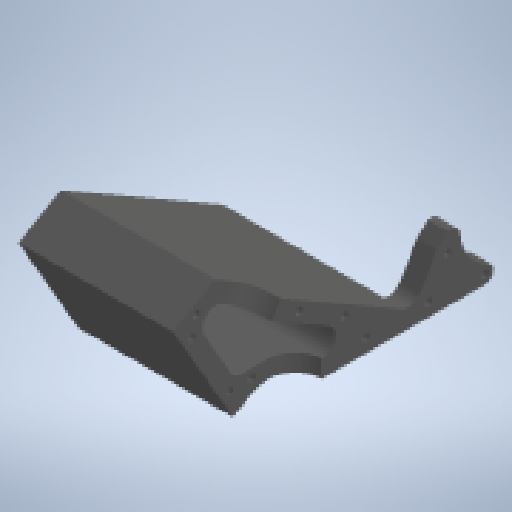
# Autodesk Inventor part: leg_upper_middle_left
Saved by Autodesk Inventor 2024.1 (Build 281209000, 209)
## iProperties
Created: 2024-10-11
Part Number: leg_upper_middle_left
Material: 一般
Document SubType Name: Modeling
Designer: hibik
Density: 1 g/cm^3
Appearance: 既定
Author: hibik
Autodesk Inventor part; units mm, degrees
ref_plane "YZ Plane" through (0, 0, 0) normal (1, 0, 0) x (0, 1, 0)
ref_plane "XZ Plane" through (0, 0, 0) normal (0, 1, 0) x (-1, 0, 0)
ref_plane "XY Plane" through (0, 0, 0) normal (0, 0, 1) x (1, 0, 0)
sketch "スケッチ1" plane through (0, 0, 0) normal (1, 0, 0) x (0, 1, 0)
  line L0 (27, 0) -> (0, 0)
  line L1 (0, 0) -> (0, -65.8723)
  line L2 (0, -65.8723) -> (27, -65.8723)
  line L3 (27, -65.8723) -> (27, -2.1436)
  line L4 (25.9282, 1.8564) -> (7.2963, 34.1277)
  line L5 (7.2963, 34.1277) -> (-16.0863, 20.6277)
  line L6 (-16.0863, 20.6277) -> (0, -7.2346)
  line L7 (0, 19.7654) -> (-4.395, 27.3777)
  circle A0 centre (0, 19.7654) radius 4.25
  circle A1 centre (13.5, -57.0823) radius 4.25
  line L8 (13.5, -65.8723) -> (13.5, -57.0823)
  circle A2 centre (0, 19.7654) radius 13.5
  circle A3 centre (13.5, -57.0823) radius 13.5
  circle A4 centre (0, 19.7654) radius 6
  circle A5 centre (13.5, -57.0823) radius 6
  circle A6 centre (-3, 24.9615) radius 1
  circle A7 centre (-5.7956, 21.3183) radius 1
  circle A8 centre (-5.1962, 16.7654) radius 1
  circle A9 centre (-1.5529, 13.9698) radius 1
  circle A10 centre (3, 14.5692) radius 1
  circle A11 centre (5.7956, 18.2125) radius 1
  circle A12 centre (13.5, -63.0823) radius 1
  circle A13 centre (17.7426, -61.3249) radius 1
  circle A14 centre (19.5, -57.0823) radius 1
  circle A15 centre (17.7426, -52.8396) radius 1
  circle A16 centre (13.5, -51.0823) radius 1
  circle A17 centre (9.2574, -52.8396) radius 1
  circle A18 centre (7.5, -57.0823) radius 1
  circle A19 centre (9.2574, -61.3249) radius 1
  circle A20 centre (5.1962, 22.7654) radius 1
  circle A21 centre (1.5529, 25.5609) radius 1
  line L9 (13.5, -57.0823) -> (50.1936, 6.4729)
  line L10 (13.5, -57.0823) -> (5.7058, -52.5823)
  line L11 (12.2058, -41.3239) -> (-0.7942, -63.8406)
  line L12 (12.2058, -41.3239) -> (3.1125, -36.0739)
  line L13 (3.1125, -36.0739) -> (27, 5.3004)
  line L14 (19.9413, 12.226) -> (-3.4413, -1.274)
  line L15 (3.1125, -36.0739) -> (0, -36.0739)
  arc A22 (27, -2.1436) -> (25.9282, 1.8564) centre (19, -2.1436) ccw
  point P0 (-14.7211, 28.9596)
  point P1 (-3.0298, -41.1381)
  point P2 (23.9702, -41.1381)
  point P3 (8.6616, 42.4596)
  point P4 (25.4699, 2.6502)
  point P5 (0, -57.0823)
  point P6 (10.7369, -43.8681)
  dimension "d11" = 12
  dimension "d12" = 12
  dimension "d4" = 27
  dimension "d5" = 150
  dimension "d6" = 27
  dimension "d7" = 8.79
  dimension "d8" = 100
  dimension "d9" = 8.79
  dimension "d10" = 8.5
  dimension "d13" = 2
  dimension "d14" = 360
  dimension "d15" = 2
  dimension "d16" = 360
  dimension "d17" = 39.4073
  dimension "d18" = 9
  dimension "d19" = 13
  dimension "d20" = 30
  dimension "d22" = 19.5
  dimension "d24" = 16.5
  dimension "d28" = 8
  constraints: 32 end point, 21 centre point, 9 perpendicular, 9 point on line, 8 coincident, 4 tangent, 3 midpoint, 2 parallel, 2 point on circle, 2 vertical alignment, 1 equal radius, 1 horizontal, 1 vertical, 40 other
  measures "d4" distance of L1.end L2.end
  measures "d5" angle of L3 L4
  measures "d6" distance between parallel lines of L6 L4
  measures "d7" distance from line of L5 L7.start
  measures "d8" distance from line of L2 L4.end
  measures "d9" distance of L8.start point (13.5, -57.082)
  measures "d10" diameter of A0
  measures "d13" diameter of A6
  measures "d15" diameter of A12
  measures "d17" distance from line of L0.start L5
  measures "d18" distance from line of L10.end L9
  measures "d19" distance from line of L11.start L10
  measures "d20" angle of L3 L9
  measures "d22" distance from line of L13 L8.end
  measures "d24" distance from line of L14 L7.start
  measures "d28" radius of A22
extrude "押し出し1" add sketch "スケッチ1" along normal blind 35 contours L13 L15 L1 L0 | L0 L1 L6 L14 L4 L13
fillet "フィレット1" radius 8 1 edges at (17.5, 0, -7.2346)
sketch "スケッチ2" plane through (35, 0, 0) normal (1, 0, 0) x (0, 0, -1)
  line L0 (21.5464, 11.5) -> (9.5919, 18.4019) projected
  arc A0 (11.0919, 24) -> (9.5919, 18.4019) centre (11.0919, 21) ccw projected
  line L1 (11.0919, 24) -> (27.0312, 24) projected
  arc A1 (29.6293, 19.5) -> (27.0312, 24) centre (27.0312, 21) ccw projected
  line L2 (29.6293, 19.5) -> (25.6444, 12.5981) projected
  arc A2 (21.5464, 11.5) -> (25.6444, 12.5981) centre (23.0464, 14.0981) ccw projected
  line L3 (-15.2943, 14.7058) -> (-13.324, 15.8433) projected
  arc A3 (-9.226, 14.7452) -> (-13.324, 15.8433) centre (-11.824, 13.2452) ccw projected
  line L4 (-9.226, 14.7452) -> (-1.726, 1.7548) projected
  arc A4 (-2.824, -2.3433) -> (-1.726, 1.7548) centre (-4.324, 0.2548) ccw projected
  line L5 (-2.824, -2.3433) -> (-4.7943, -3.4808) projected
  arc A5 (-9.2878, -0.6865) -> (-4.7943, -3.4808) centre (-6.2943, -0.8827) ccw projected
  arc A6 (-9.2878, -0.6865) -> (-15.1212, 9.4171) centre (-19.7654, 0) ccw projected
  arc A7 (-15.2943, 14.7058) -> (-15.1212, 9.4171) centre (-13.7943, 12.1077) ccw projected
  line L6 (45.8573, 3) -> (37.0726, 3) projected
  arc A8 (35.5726, 3.4019) -> (37.0726, 3) centre (37.0726, 6) ccw projected
  line L7 (35.5726, 3.4019) -> (31.9387, 5.5) projected
  arc A9 (30.8406, 9.5981) -> (31.9387, 5.5) centre (33.4387, 8.0981) ccw projected
  line L8 (30.8406, 9.5981) -> (38.2895, 22.5) projected
  arc A10 (40.8876, 24) -> (38.2895, 22.5) centre (40.8876, 21) ccw projected
  line L9 (40.8876, 24) -> (45.8573, 24) projected
  arc A11 (48.3517, 19.3333) -> (45.8573, 24) centre (45.8573, 21) ccw projected
  arc A12 (48.3517, 19.3333) -> (48.3517, 7.6667) centre (57.0823, 13.5) ccw projected
  arc A13 (45.8573, 3) -> (48.3517, 7.6667) centre (45.8573, 6) ccw projected
  line L10 (-1.1502, 19.9851) -> (16.8406, 9.5981) projected
  arc A14 (15.3406, 4) -> (16.8406, 9.5981) centre (15.3406, 7) ccw projected
  line L11 (15.3406, 4) -> (3.3286, 4) projected
  arc A15 (0.7306, 5.5) -> (3.3286, 4) centre (3.3286, 7) ccw projected
  line L12 (0.7306, 5.5) -> (-5.2619, 15.8792) projected
  arc A16 (-4.1638, 19.9772) -> (-5.2619, 15.8792) centre (-2.6638, 17.3792) ccw projected
  line L13 (-4.1638, 19.9772) -> (-4.1502, 19.9851) projected
  arc A17 (-1.1502, 19.9851) -> (-4.1502, 19.9851) centre (-2.6502, 17.387) ccw projected
  arc A18 (57.3667, 17.7405) -> (59.3483, 18.9706) centre (57.5005, 19.736) ccw projected
  line L14 (59.3483, 18.9706) -> (59.8105, 20.0866) projected
  arc A19 (59.8105, 20.0866) -> (55.1911, 27) centre (55.1911, 22) ccw projected
  line L15 (55.1911, 27) -> (2.1436, 27) projected
  arc A20 (2.1436, 27) -> (-1.8564, 25.9282) centre (2.1436, 19) ccw projected
  line L16 (-1.8564, 25.9282) -> (-24.8776, 12.6369) projected
  arc A21 (-24.8776, 12.6369) -> (-25.4214, 4.34) centre (-22.3776, 8.3068) ccw projected
  line L17 (-25.4214, 4.34) -> (-24.4631, 3.6047) projected
  arc A22 (-24.4631, 3.6047) -> (-22.1319, 3.5302) centre (-23.2456, 5.1914) ccw projected
  arc A23 (-17.8914, -3.8146) -> (-22.1319, 3.5302) centre (-19.7654, 0) ccw projected
  arc A24 (-17.8914, -3.8146) -> (-18.9925, -5.8707) centre (-17.0096, -5.6096) ccw projected
  line L18 (-18.9925, -5.8707) -> (-18.8348, -7.0683) projected
  arc A25 (-18.8348, -7.0683) -> (-11.3776, -10.7458) centre (-13.8776, -6.4156) ccw projected
  line L19 (-11.3776, -10.7458) -> (5.3782, -1.0718) projected
  arc A26 (9.3782, 0) -> (5.3782, -1.0718) centre (9.3782, -8) ccw projected
  line L20 (9.3782, 0) -> (55.1911, 0) projected
  arc A27 (55.1911, 0) -> (59.8105, 6.9134) centre (55.1911, 5) ccw projected
  line L21 (59.8105, 6.9134) -> (59.3483, 8.0294) projected
  arc A28 (59.3483, 8.0294) -> (57.3667, 9.2595) centre (57.5005, 7.264) ccw projected
  arc A29 (57.3667, 17.7405) -> (57.3667, 9.2595) centre (57.0823, 13.5) ccw projected
  circle A30 centre (-22.7654, 5.1962) radius 1 projected
  circle A31 centre (-18.2125, 5.7956) radius 1 projected
  circle A32 centre (-14.5692, 3) radius 1 projected
  circle A33 centre (-13.9698, -1.5529) radius 1 projected
  circle A34 centre (-16.7654, -5.1962) radius 1 projected
  circle A35 centre (57.0823, 19.5) radius 1 projected
  circle A36 centre (52.8396, 17.7426) radius 1 projected
  circle A37 centre (51.0823, 13.5) radius 1 projected
  circle A38 centre (52.8396, 9.2574) radius 1 projected
  circle A39 centre (57.0823, 7.5) radius 1 projected
  circle A40 centre (5.5061, 2) radius 1 projected
  circle A41 centre (10.1981, 15.7425) radius 1 projected
  circle A42 centre (25.3406, 3) radius 1 projected
  circle A43 centre (0.5061, 1.8888) radius 1 projected
  circle A44 centre (20.5464, 9.7679) radius 1 projected
  circle A45 centre (-7.9939, 16.6112) radius 1 projected
  circle A46 centre (-6.8958, 20.7093) radius 1 projected
  point P0 (0, 0)
extrude "押し出し2" cut sketch "スケッチ2" against normal through all contours L10 A14 L11 A15 L12 A16 L13 A17
sketch "スケッチ3" plane through (0, 0, 0) normal (-1, 0, 0) x (0, 0, 1)
  arc A0 (-3.3286, 4) -> (-0.7306, 5.5) centre (-3.3286, 7) ccw projected
  line L0 (-3.3286, 4) -> (-15.3406, 4) projected
  arc A1 (-16.8406, 9.5981) -> (-15.3406, 4) centre (-15.3406, 7) ccw projected
  line L1 (-16.8406, 9.5981) -> (1.1502, 19.9851) projected
  arc A2 (4.1502, 19.9851) -> (1.1502, 19.9851) centre (2.6502, 17.387) ccw projected
  line L2 (4.1502, 19.9851) -> (4.1638, 19.9772) projected
  arc A3 (5.2619, 15.8792) -> (4.1638, 19.9772) centre (2.6638, 17.3792) ccw projected
  line L3 (5.2619, 15.8792) -> (-0.7306, 5.5) projected
  line L4 (-36.0739, 3.1125) -> (2.6502, 25.4699) projected
  line L5 (-36.0739, 0) -> (-36.0739, 3.1125) projected
  line L6 (-9.3782, 0) -> (-36.0739, 0) projected
  arc A4 (-5.3782, -1.0718) -> (-9.3782, 0) centre (-9.3782, -8) ccw projected
  line L7 (-1.274, -3.4413) -> (-5.3782, -1.0718) projected
  line L8 (12.226, 19.9413) -> (-1.274, -3.4413) projected
  line L9 (2.6502, 25.4699) -> (12.226, 19.9413) projected
  line L10 (1.1502, 19.9851) -> (-0.8498, 23.4492)
  line L11 (-6.0459, 20.4492) -> (-4.0459, 16.9851)
  line L12 (-15.3346, 4) -> (-15.3346, 0)
  line L13 (-3.3286, 4) -> (-15.3406, 4) projected
  line L14 (-9.3782, 0) -> (-9.3782, 4)
  point P0 (0, 0)
  point P1 (-9.3346, 4)
  dimension "d33" = 6
  dimension "d34" = 6
  constraints: 8 end point, 6 point on line, 4 perpendicular, 1 midpoint
  measures "d33" distance between parallel lines of L10 L11
  measures "d34" distance from line of point (-9.335, 4) L12
extrude "押し出し3" add sketch "スケッチ3" along normal blind 6 contours L12 L6 L5 L4 L11 L1 A1 L0
fillet "フィレット2" radius 6 2 edges at (0, 18.7171, -5.0459) (0, 2, -15.3346)
sketch "スケッチ4" plane through (-6, 0, 0) normal (-1, 0, 0) x (0, 0, 1)
  arc A0 (-39.4731, 0) -> (-36.875, 4.5) centre (-39.4731, 3) ccw projected
  line L0 (-39.4731, 0) -> (-55.1911, 0) projected
  arc A1 (-59.8105, 6.9134) -> (-55.1911, 0) centre (-55.1911, 5) ccw projected
  line L1 (-59.8105, 6.9134) -> (-59.3483, 8.0294) projected
  arc A2 (-57.3667, 9.2595) -> (-59.3483, 8.0294) centre (-57.5005, 7.264) ccw projected
  arc A3 (-57.3667, 9.2595) -> (-57.3667, 17.7405) centre (-57.0823, 13.5) ccw projected
  arc A4 (-59.3483, 18.9706) -> (-57.3667, 17.7405) centre (-57.5005, 19.736) ccw projected
  line L2 (-59.3483, 18.9706) -> (-59.7128, 19.8506) projected
  arc A5 (-56.8847, 23.9981) -> (-59.7128, 19.8506) centre (-56.9411, 20.9987) ccw projected
  arc A6 (-49.4902, 20.7534) -> (-56.8847, 23.9981) centre (-57.0823, 13.5) ccw projected
  line L3 (-49.4902, 20.7534) -> (-41.5728, 12.4662) projected
  arc A7 (-41.1438, 11.8938) -> (-41.5728, 12.4662) centre (-43.7419, 10.3938) ccw projected
  line L4 (-41.1438, 11.8938) -> (-36.875, 4.5) projected
  circle A8 centre (-57.0823, 19.5) radius 1 projected
  circle A9 centre (-52.8396, 17.7426) radius 1 projected
  circle A10 centre (-51.0823, 13.5) radius 1 projected
  circle A11 centre (-52.8396, 9.2574) radius 1 projected
  circle A12 centre (-57.0823, 7.5) radius 1 projected
  circle A13 centre (-57.0823, 13.5) radius 10.5
  arc A14 (-50.4826, 5.3333) -> (-46.6014, 12.8657) centre (-57.0823, 13.5) ccw projected
  arc A15 (-44.6051, 14.7449) -> (-46.6014, 12.8657) centre (-44.6051, 12.7449) ccw projected
  arc A16 (-52.9671, 3.84) -> (-46.6014, 12.8657) centre (-57.0823, 13.5) ccw projected
  arc A17 (-52.9671, 3.84) -> (-52.1833, 0) centre (-52.1833, 2) ccw projected
  line L5 (-15.3782, 0) -> (-52.1833, 0) projected
  line L6 (-15.3782, 0) -> (-15.3782, 4.0002) projected
  arc A18 (-16.8406, 9.5981) -> (-15.3782, 4.0002) centre (-15.3406, 7) ccw projected
  line L7 (-16.8406, 9.5981) -> (-4.0459, 16.9851) projected
  line L8 (-4.0459, 16.9851) -> (-6.0459, 20.4492) projected
  line L9 (-6.0459, 20.4492) -> (-15.926, 14.7449) projected
  line L10 (-15.926, 14.7449) -> (-44.6051, 14.7449) projected
  line L11 (-36.3155, 12.5308) -> (-30.9571, 12.5308) projected
  arc A19 (-29.4571, 6.9328) -> (-30.9571, 12.5308) centre (-30.9571, 9.5308) ccw projected
  line L12 (-29.4571, 6.9328) -> (-33.4759, 4.6125) projected
  arc A20 (-37.5739, 5.7106) -> (-33.4759, 4.6125) centre (-34.9759, 7.2106) ccw projected
  line L13 (-37.5739, 5.7106) -> (-38.9135, 8.0308) projected
  arc A21 (-36.3155, 12.5308) -> (-38.9135, 8.0308) centre (-36.3155, 9.5308) ccw projected
  arc A22 (-44.6051, 14.7449) -> (-46.6014, 12.8657) centre (-44.6051, 12.7449) ccw projected
  arc A23 (-52.9671, 3.84) -> (-46.6014, 12.8657) centre (-57.0823, 13.5) ccw projected
  arc A24 (-52.9671, 3.84) -> (-52.1833, 0) centre (-52.1833, 2) ccw projected
  line L14 (-15.3782, 0) -> (-52.1833, 0) projected
  line L15 (-15.3782, 0) -> (-15.3782, 4.0002) projected
  arc A25 (-16.8406, 9.5981) -> (-15.3782, 4.0002) centre (-15.3406, 7) ccw projected
  line L16 (-16.8406, 9.5981) -> (-4.0459, 16.9851) projected
  line L17 (-4.0459, 16.9851) -> (-6.0459, 20.4492) projected
  line L18 (-6.0459, 20.4492) -> (-15.926, 14.7449) projected
  line L19 (-15.926, 14.7449) -> (-44.6051, 14.7449) projected
  line L20 (-36.3155, 12.5308) -> (-30.9571, 12.5308) projected
  arc A26 (-29.4571, 6.9328) -> (-30.9571, 12.5308) centre (-30.9571, 9.5308) ccw projected
  line L21 (-29.4571, 6.9328) -> (-33.4759, 4.6125) projected
  arc A27 (-37.5739, 5.7106) -> (-33.4759, 4.6125) centre (-34.9759, 7.2106) ccw projected
  line L22 (-37.5739, 5.7106) -> (-38.9135, 8.0308) projected
  arc A28 (-36.3155, 12.5308) -> (-38.9135, 8.0308) centre (-36.3155, 9.5308) ccw projected
  line L23 (-6.0459, 20.4492) -> (-36.0739, 3.1125) projected
  line L24 (-36.0739, 3.1125) -> (-36.0739, 0) projected
  circle A29 centre (-52.1833, 2) radius 1 projected
  circle A30 centre (-39.4731, 3) radius 1 projected
  circle A31 centre (-43.7419, 10.3938) radius 1 projected
  circle A32 centre (-10.1981, 15.7425) radius 1 projected
  circle A33 centre (-20.5464, 9.7679) radius 1 projected
  circle A34 centre (-25.3406, 3) radius 1 projected
  circle A35 centre (-52.1833, 2) radius 1 projected
  circle A36 centre (-39.4731, 3) radius 1 projected
  circle A37 centre (-43.7419, 10.3938) radius 1 projected
  circle A38 centre (-10.1981, 15.7425) radius 1 projected
  circle A39 centre (-20.5464, 9.7679) radius 1 projected
  circle A40 centre (-25.3406, 3) radius 1 projected
  point P0 (-48.6288, 19.8517)
  point P1 (-56.8847, 23.9981)
  point P2 (-59.9256, 3.3923)
  point P3 (-56.8847, 23.9981)
  point P4 (-43.7498, 14.7449)
  point P5 (-46.6012, 12.8697)
  point P6 (-52.9703, 3.8386)
  point P7 (-37.5718, 5.7069)
  point P8 (-39.4697, 0)
  constraints: 1 centre point, 1 coincident, 1 tangent
ref_plane "作業平面1" through (-1.5, -10.2702, -70.5828) normal (-1, 0, 0) x (0, 0, 1)
extrude "押し出し4" add sketch "スケッチ4" against normal up to surface (4.5 mm away) contours L0 A17 A13 A15 L10 L3 A7 L4 A0 | A0 L4 A20 L23 L24 L5 | A29 | A30 | A31
sketch "スケッチ5" plane through (35, 0, 0) normal (1, 0, 0) x (0, 0, -1)
  line L0 (36.0739, 3.1125) -> (-2.6502, 25.4699) projected
  circle A0 centre (5.5061, 2) radius 1 construction
  circle A1 centre (10.1981, 15.7425) radius 1 construction
  circle A2 centre (25.3406, 3) radius 1 construction
  circle A3 centre (0.5061, 1.8888) radius 1 construction
  circle A4 centre (20.5464, 9.7679) radius 1 construction
  circle A5 centre (-7.9939, 16.6112) radius 1 construction
  circle A6 centre (-6.8958, 20.7093) radius 1 construction
  line L1 (21.5464, 11.5) -> (9.5919, 18.4019) projected
  arc A7 (11.0919, 24) -> (9.5919, 18.4019) centre (11.0919, 21) ccw projected
  line L2 (11.0919, 24) -> (27.0312, 24) projected
  arc A8 (29.6293, 19.5) -> (27.0312, 24) centre (27.0312, 21) ccw projected
  line L3 (29.6293, 19.5) -> (25.6444, 12.5981) projected
  arc A9 (21.5464, 11.5) -> (25.6444, 12.5981) centre (23.0464, 14.0981) ccw projected
  line L4 (-15.2943, 14.7058) -> (-13.324, 15.8433) projected
  arc A10 (-9.226, 14.7452) -> (-13.324, 15.8433) centre (-11.824, 13.2452) ccw projected
  line L5 (-9.226, 14.7452) -> (-1.726, 1.7548) projected
  arc A11 (-2.824, -2.3433) -> (-1.726, 1.7548) centre (-4.324, 0.2548) ccw projected
  line L6 (-2.824, -2.3433) -> (-4.7943, -3.4808) projected
  arc A12 (-9.2878, -0.6865) -> (-4.7943, -3.4808) centre (-6.2943, -0.8827) ccw projected
  arc A13 (-9.2878, -0.6865) -> (-15.1212, 9.4171) centre (-19.7654, 0) ccw projected
  arc A14 (-15.2943, 14.7058) -> (-15.1212, 9.4171) centre (-13.7943, 12.1077) ccw projected
  line L7 (45.8573, 3) -> (37.0726, 3) projected
  arc A15 (35.5726, 3.4019) -> (37.0726, 3) centre (37.0726, 6) ccw projected
  line L8 (35.5726, 3.4019) -> (31.9387, 5.5) projected
  arc A16 (30.8406, 9.5981) -> (31.9387, 5.5) centre (33.4387, 8.0981) ccw projected
  line L9 (30.8406, 9.5981) -> (38.2895, 22.5) projected
  arc A17 (40.8876, 24) -> (38.2895, 22.5) centre (40.8876, 21) ccw projected
  line L10 (40.8876, 24) -> (45.8573, 24) projected
  arc A18 (48.3517, 19.3333) -> (45.8573, 24) centre (45.8573, 21) ccw projected
  arc A19 (48.3517, 19.3333) -> (48.3517, 7.6667) centre (57.0823, 13.5) ccw projected
  arc A20 (45.8573, 3) -> (48.3517, 7.6667) centre (45.8573, 6) ccw projected
  line L11 (-1.1502, 19.9851) -> (16.8406, 9.5981) projected
  arc A21 (15.3406, 4) -> (16.8406, 9.5981) centre (15.3406, 7) ccw projected
  line L12 (15.3406, 4) -> (3.3286, 4) projected
  arc A22 (0.7306, 5.5) -> (3.3286, 4) centre (3.3286, 7) ccw projected
  line L13 (0.7306, 5.5) -> (-5.2619, 15.8792) projected
  arc A23 (-4.1638, 19.9772) -> (-5.2619, 15.8792) centre (-2.6638, 17.3792) ccw projected
  line L14 (-4.1638, 19.9772) -> (-4.1502, 19.9851) projected
  arc A24 (-1.1502, 19.9851) -> (-4.1502, 19.9851) centre (-2.6502, 17.387) ccw projected
  arc A25 (57.3667, 17.7405) -> (59.3483, 18.9706) centre (57.5005, 19.736) ccw projected
  line L15 (59.3483, 18.9706) -> (59.8105, 20.0866) projected
  arc A26 (59.8105, 20.0866) -> (55.1911, 27) centre (55.1911, 22) ccw projected
  line L16 (55.1911, 27) -> (2.1436, 27) projected
  arc A27 (2.1436, 27) -> (-1.8564, 25.9282) centre (2.1436, 19) ccw projected
  line L17 (-1.8564, 25.9282) -> (-24.8776, 12.6369) projected
  arc A28 (-24.8776, 12.6369) -> (-25.4214, 4.34) centre (-22.3776, 8.3068) ccw projected
  line L18 (-25.4214, 4.34) -> (-24.4631, 3.6047) projected
  arc A29 (-24.4631, 3.6047) -> (-22.1319, 3.5302) centre (-23.2456, 5.1914) ccw projected
  arc A30 (-17.8914, -3.8146) -> (-22.1319, 3.5302) centre (-19.7654, 0) ccw projected
  arc A31 (-17.8914, -3.8146) -> (-18.9925, -5.8707) centre (-17.0096, -5.6096) ccw projected
  line L19 (-18.9925, -5.8707) -> (-18.8348, -7.0683) projected
  arc A32 (-18.8348, -7.0683) -> (-11.3776, -10.7458) centre (-13.8776, -6.4156) ccw projected
  line L20 (-11.3776, -10.7458) -> (5.3782, -1.0718) projected
  arc A33 (9.3782, 0) -> (5.3782, -1.0718) centre (9.3782, -8) ccw projected
  line L21 (9.3782, 0) -> (55.1911, 0) projected
  arc A34 (55.1911, 0) -> (59.8105, 6.9134) centre (55.1911, 5) ccw projected
  line L22 (59.8105, 6.9134) -> (59.3483, 8.0294) projected
  arc A35 (59.3483, 8.0294) -> (57.3667, 9.2595) centre (57.5005, 7.264) ccw projected
  arc A36 (57.3667, 17.7405) -> (57.3667, 9.2595) centre (57.0823, 13.5) ccw projected
  circle A37 centre (-22.7654, 5.1962) radius 1 projected
  circle A38 centre (-18.2125, 5.7956) radius 1 projected
  circle A39 centre (-14.5692, 3) radius 1 projected
  circle A40 centre (-13.9698, -1.5529) radius 1 projected
  circle A41 centre (-16.7654, -5.1962) radius 1 projected
  circle A42 centre (57.0823, 19.5) radius 1 projected
  circle A43 centre (52.8396, 17.7426) radius 1 projected
  circle A44 centre (51.0823, 13.5) radius 1 projected
  circle A45 centre (52.8396, 9.2574) radius 1 projected
  circle A46 centre (57.0823, 7.5) radius 1 projected
  circle A47 centre (-6.8958, 20.7093) radius 0.8
  circle A48 centre (-7.9939, 16.6112) radius 0.8
  circle A49 centre (0.5061, 1.8888) radius 0.8
  circle A50 centre (5.5061, 2) radius 0.8
  circle A51 centre (25.3406, 3) radius 0.8
  circle A52 centre (20.5464, 9.7679) radius 0.8
  circle A53 centre (10.1981, 15.7425) radius 0.8
  point P0 (0, 0)
  dimension "d42" = 1.6
  constraints: 7 centre point, 7 coincident, 6 equal radius
  measures "d42" diameter of A47
extrude "押し出し5" cut sketch "スケッチ5" against normal through all contours A47 | A48 | A49 | A50 | A51 | A52 | A53
sketch "スケッチ6" plane through (-6, 0, 0) normal (-1, 0, 0) x (0, 0, 1)
  circle A0 centre (-43.7419, 10.3938) radius 1 construction
  circle A1 centre (-39.4731, 3) radius 1 construction
  circle A2 centre (-52.1833, 2) radius 1 construction
  circle A3 centre (-43.7419, 10.3938) radius 0.8
  circle A4 centre (-39.4731, 3) radius 0.8
  circle A5 centre (-52.1833, 2) radius 0.8
  point P0 (0, 0)
  dimension "d43" = 1.6
  dimension "d44" = 1.6
  dimension "d45" = 1.6
  constraints: 3 centre point, 3 coincident
  measures "d43" diameter of A3
  measures "d44" diameter of A4
  measures "d45" diameter of A5
extrude "押し出し6" cut sketch "スケッチ6" against normal through all
mirror "ミラー1" about plane through (0, 0, 0) normal (1, 0, 0) remove original yes
fillet "フィレット4" radius 2.4 2 edges at (-16.75, 3.1125, -36.0739) (-16.75, 0, -36.0739)
